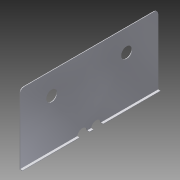
# Autodesk Inventor part: Fin_narrow
Saved by Autodesk Inventor 2015 (Build 190159000, 159)
## iProperties
Created: 2015-08-21
Part Number: Fin_narrow
Material: Aluminum 6061
Document SubType Name: Modeling
Designer: Kyle
Density: 2.7 g/cm^3
Appearance: Aluminum - Flat
Author: Kyle
Autodesk Inventor part; units mm, degrees
ref_plane "YZ Plane" through (0, 0, 0) normal (1, 0, 0) x (0, 1, 0)
ref_plane "XZ Plane" through (0, 0, 0) normal (0, 1, 0) x (-1, 0, 0)
ref_plane "XY Plane" through (0, 0, 0) normal (0, 0, 1) x (1, 0, 0)
sketch "Sketch1" plane through (0, 0, 0) normal (0, 0, 1) x (1, 0, 0)
  line L0 (0, 0) -> (1.8311, 0)
  line L1 (0, 0) -> (0, 45.085)
  line L2 (0.381, 45.085) -> (0.381, 0.381)
  line L3 (0.381, 0.381) -> (1.8311, 0.381)
  line L4 (1.8311, 0.381) -> (1.8311, 0)
  line L5 (0.381, 45.085) -> (0, 45.085)
  dimension "d0" = 1.8311
  dimension "d1" = 45.085
  dimension "d2" = 0.381
  constraints: 12 end point, 2 vertical, 1 horizontal, 1 perpendicular, 1 other
  measures "d0" distance of L0.start L0.end
  measures "d1" distance of L0.start L1.end
  measures "d2" distance between parallel lines of L1 L2
extrude "Extrusion1" add sketch "Sketch1" along normal blind 88.9
fillet "Fillet1" radius 2.54 2 edges at (0.1905, 45.085, 88.9) (0.1905, 45.085, 0)
sketch "Sketch2" plane through (0, 0, 0) normal (-1, 0, 0) x (0, 0, 1)
  line L0 (0, 0) -> (88.9, 0) projected
  circle A0 centre (40.005, 0) radius 3.175
  circle A1 centre (48.895, 0) radius 3.2307
  dimension "d6" = 6.35
  dimension "d7" = 8.89
  dimension "d8" = 40.005
  constraints: 2 centre point, 2 point on line
  measures "d6" diameter of A0
  measures "d7" distance of A0.centre A1.centre
  measures "d8" distance of L0.end A1.centre
extrude "Extrusion2" cut sketch "Sketch2" against normal blind 88.9
sketch "Sketch3" plane through (0, 0, 0) normal (-1, 0, 0) x (0, 0, 1)
  circle A0 centre (20.32, 31.115) radius 3.4925
  circle A1 centre (68.58, 31.115) radius 3.4925
  line L0 (88.9, 42.545) -> (88.9, 0) projected
  line L1 (0, 42.545) -> (0, 0) projected
  line L2 (2.54, 45.085) -> (86.36, 45.085) projected
  dimension "d11" = 6.985
  dimension "d12" = 6.985
  dimension "d13" = 20.32
  dimension "d14" = 20.32
  dimension "d15" = 13.97
  dimension "d16" = 13.97
  constraints: 2 centre point
  measures "d11" diameter of A0
  measures "d12" diameter of A1
  measures "d13" distance from line of L0 A1.centre
  measures "d14" distance from line of L1 A0.centre
  measures "d15" distance from line of L2 A0.centre
  measures "d16" distance from line of L2 A1.centre
extrude "Extrusion3" cut sketch "Sketch3" against normal blind 88.9
body "Solid1"
